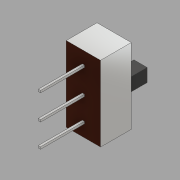
# Autodesk Inventor part: switch small
Saved by Autodesk Inventor 2018 (Build 220112000, 112)
## iProperties
Created: 2018-07-02
Part Number: switch small
Material: Generic
Document SubType Name: Modeling
Designer: adams
Density: 1 g/cm^3
Appearance: Aluminum - Polished
Author: adams
Autodesk Inventor part; units mm, degrees
ref_plane "YZ Plane" through (0, 0, 0) normal (1, 0, 0) x (0, 1, 0)
ref_plane "XZ Plane" through (0, 0, 0) normal (0, 1, 0) x (-1, 0, 0)
ref_plane "XY Plane" through (0, 0, 0) normal (0, 0, 1) x (1, 0, 0)
sketch "Sketch1" plane through (0, 0, 0) normal (0, 1, 0) x (-1, 0, 0)
  line L0 (0, 0) -> (-3.9, 0)
  line L1 (-3.9, 0) -> (-3.9, -8.55)
  line L2 (-3.9, -8.55) -> (0, -8.55)
  line L3 (0, -8.55) -> (0, 0)
  dimension "d0" = 3.9
  dimension "d1" = 8.55
  constraints: 8 end point, 2 parallel, 1 horizontal, 1 perpendicular
  measures "d0" distance of L2.end L1.end
  measures "d1" distance of L1.end L0.end
extrude "Extrusion1" add sketch "Sketch1" along normal blind 3.5
sketch "Sketch2" plane through (0, 3.5, 0) normal (0, 1, 0) x (1, 0, 0)
  line L0 (0, 8.55) -> (0, 0) projected
  line L1 (3.9, 0) -> (3.9, 8.55) projected
  line L2 (0, 0) -> (3.9, 0)
  line L3 (3.9, 0) -> (3.9, 8.55)
  line L4 (3.9, 8.55) -> (0, 8.55)
  line L5 (0, 8.55) -> (0, 0)
  line L6 (1.95, 8.55) -> (1.95, 6.05) construction
  line L7 (1.95, 0) -> (1.95, 2.5) construction
  line L8 (1.95, 0) -> (4.45, 0) construction
  line L9 (0, 4.275) -> (1.7, 4.275) construction
  line L10 (0, 4.275) -> (1.7, 4.275) construction
  line L11 (3.9, 4.275) -> (2.2, 4.275) construction
  line L12 (3.9, 4.275) -> (5.6, 4.275) construction
  line L13 (2.2, 2.5) -> (1.7, 2.5)
  line L14 (1.7, 6.05) -> (2.2, 6.05)
  line L15 (2.2, 2.5) -> (1.7, 6.05) construction
  line L16 (1.7, 2.5) -> (2.2, 6.05) construction
  line L17 (1.7, 2.5) -> (1.2, 2.5)
  line L18 (1.7, 2.5) -> (2.2, 2.5) construction
  line L19 (2.2, 2.5) -> (2.7, 2.5)
  line L20 (2.2, 2.5) -> (2.7, 2.5) construction
  line L21 (2.7, 2.5) -> (2.7, 6.05)
  line L22 (2.7, 6.05) -> (1.2, 6.05)
  line L23 (1.2, 6.05) -> (1.2, 2.5)
  line L24 (1.2, 2.5) -> (2.7, 2.5)
  line L25 (2.7, 2.5) -> (2.7, 6.05)
  line L26 (2.7, 6.05) -> (1.2, 6.05)
  line L27 (1.2, 6.05) -> (1.2, 2.5)
  point P0 (1.95, 4.275)
  dimension "d4" = 2.5
  dimension "d5" = 2.5
  dimension "d6" = 90
  dimension "d7" = 1.7
  dimension "d8" = 0
  dimension "d9" = 1.7
  dimension "d10" = 180
  dimension "d13" = 0.5
  dimension "d14" = 0.5
  dimension "d15" = 180
  dimension "d16" = 0.5
  dimension "d17" = 0
  constraints: 52 end point, 11 equal length, 11 horizontal, 6 midpoint, 5 perpendicular, 2 vertical
  measures "d4" distance of L6.start L6.end
  measures "d5" distance of L7.start L7.end
  measures "d6" angle of L8 L7
  measures "d7" distance of L9.start L9.end
  measures "d8" distance between parallel lines of L9 L10
  measures "d9" distance of L11.start L11.end
  measures "d10" angle of L11 L12
  measures "d13" distance of L13.start L13.end
  measures "d14" distance of L13.end L17.end
  measures "d15" angle of L17 L18
  measures "d16" distance of L18.end L19.end
  measures "d17" distance between parallel lines of L19 L20
extrude "Extrusion3" cut sketch "Sketch2" against normal blind 0.11 contours L13 L17 L23 L22 L14 L21 L19
sketch "Sketch3" plane through (0, 3.39, 0) normal (0, 1, 0) x (1, 0, 0)
  line L0 (1.2, 2.5) -> (1.2, 6.05) projected
  line L1 (1.2, 6.05) -> (2.7, 6.05)
  line L2 (2.7, 6.05) -> (2.7, 4.55)
  line L3 (2.7, 4.55) -> (1.2, 4.55)
  line L4 (1.2, 4.55) -> (1.2, 6.05)
  point P0 (0, 0)
  dimension "d20" = 1.5
  dimension "d21" = 1.5
  constraints: 8 end point, 2 parallel, 1 horizontal, 1 perpendicular
  measures "d20" distance of L2.end L3.end
  measures "d21" distance of L1.end L2.end
extrude "Extrusion4" add sketch "Sketch3" along normal blind 3.11
sketch "Sketch4" plane through (0, 0, 0) normal (0, -1, 0) x (1, 0, 0)
  line L0 (0, 0) -> (3.9, 0) projected
  line L1 (1.95, 0) -> (1.95, -1.5) construction
  line L2 (1.95, 0) -> (3.45, 0) construction
  line L3 (1.825, -1.625) -> (2.075, -1.625)
  line L4 (2.075, -1.625) -> (2.075, -1.375)
  line L5 (2.075, -1.375) -> (1.825, -1.375)
  line L6 (1.825, -1.375) -> (1.825, -1.625)
  line L7 (1.825, -1.625) -> (2.075, -1.375) construction
  line L8 (2.075, -1.625) -> (1.825, -1.375) construction
  line L9 (3.9, -8.55) -> (0, -8.55) projected
  line L10 (1.95, -8.55) -> (1.95, -7.05) construction
  line L11 (1.95, -8.55) -> (3.45, -8.55) construction
  line L12 (1.825, -7.175) -> (2.075, -7.175)
  line L13 (2.075, -7.175) -> (2.075, -6.925)
  line L14 (2.075, -6.925) -> (1.825, -6.925)
  line L15 (1.825, -6.925) -> (1.825, -7.175)
  line L16 (1.825, -7.175) -> (2.075, -6.925) construction
  line L17 (2.075, -7.175) -> (1.825, -6.925) construction
  line L18 (1.95, -1.375) -> (1.95, -4.375) construction
  line L19 (1.95, -1.375) -> (4.95, -1.375) construction
  line L20 (1.825, -4.5) -> (2.075, -4.5)
  line L21 (2.075, -4.5) -> (2.075, -4.25)
  line L22 (2.075, -4.25) -> (1.825, -4.25)
  line L23 (1.825, -4.25) -> (1.825, -4.5)
  line L24 (1.825, -4.5) -> (2.075, -4.25) construction
  line L25 (2.075, -4.5) -> (1.825, -4.25) construction
  dimension "d24" = 1.5
  dimension "d25" = 90
  dimension "d26" = 0.25
  dimension "d27" = 0.25
  dimension "d28" = 1.5
  dimension "d29" = 90
  dimension "d30" = 0.25
  dimension "d31" = 0.25
  dimension "d32" = 3
  dimension "d33" = 90
  dimension "d34" = 0.25
  dimension "d35" = 0.25
  constraints: 48 end point, 9 midpoint, 6 horizontal, 6 parallel, 6 perpendicular, 3 vertical
  measures "d24" distance of L1.start L1.end
  measures "d25" angle of L1 L2
  measures "d26" distance of L5.end L4.end
  measures "d27" distance of L4.end L3.end
  measures "d28" distance of L10.start L10.end
  measures "d29" angle of L11 L10
  measures "d30" distance of L14.end L13.end
  measures "d31" distance of L13.end L12.end
  measures "d32" distance of L18.start L18.end
  measures "d33" angle of L18 L19
  measures "d34" distance of L22.end L21.end
  measures "d35" distance of L21.end L20.end
extrude "Extrusion5" add sketch "Sketch4" along normal blind 5
body "Solid1"
